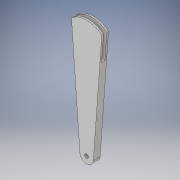
# Autodesk Inventor part: poker
Saved by Autodesk Inventor 2018 (Build 220112000, 112)
## iProperties
Created: 2017-12-11
Part Number: poker
Material: Generic
Document SubType Name: Modeling
Designer: ragna
Density: 1 g/cm^3
Appearance: Default
Author: ragna
Autodesk Inventor part; units mm, degrees
ref_plane "YZ Plane" through (0, 0, 0) normal (1, 0, 0) x (0, 1, 0)
ref_plane "XZ Plane" through (0, 0, 0) normal (0, 1, 0) x (-1, 0, 0)
ref_plane "XY Plane" through (0, 0, 0) normal (0, 0, 1) x (1, 0, 0)
sketch "Sketch1" plane through (0, 0, 0) normal (0, 0, 1) x (1, 0, 0)
  arc A0 (-0.1732, -0.9119) -> (-5.8268, -0.9119) centre (-3, -4.8375) ccw
  arc A1 (-5.8268, -1.5881) -> (-0.1732, -1.5881) centre (-3, 2.3375) ccw
  circle A2 centre (-5.5833, -1.25) radius 0.4167
  circle A3 centre (-0.4167, -1.25) radius 0.4167
  line L0 (-6, 0) -> (0, 0)
  line L1 (0, 0) -> (0, -2.5)
  line L2 (0, -2.5) -> (-6, -2.5)
  line L3 (-6, -2.5) -> (-6, 0)
  point P0 (-1.5, -3.25)
  dimension "d8" = 4.8375
  dimension "d11" = 0.8333
  dimension "d12" = 6
  dimension "d13" = 2.5
  dimension "d14" = 0.8333
  dimension "d22" = 4.8375
  constraints: 8 end point, 8 point on circle, 8 tangent, 4 centre point, 2 parallel, 1 coincident, 1 horizontal, 1 perpendicular, 1 vertical alignment
  measures "d8" radius of A0
  measures "d11" diameter of A3
  measures "d12" distance of L1.end L2.end
  measures "d13" distance of L2.end L0.start
  measures "d14" diameter of A2
  measures "d22" radius of A1
extrude "Extrusion1" add sketch "Sketch1" against normal blind 0.25 contours A3 A1 A2 A0 | A3 | A2
sketch "Sketch2" plane through (0, 0, 0) normal (0, 0, 1) x (1, 0, 0)
  arc A0 (-0.1732, -0.9119) -> (-5.8268, -0.9119) centre (-3, -4.8375) ccw projected
  arc A1 (1.5, 0.3105) -> (-7.5, 0.3105) centre (-3, -4.8375) ccw
  line L0 (-4.9944, -33.1493) -> (-7.5, 0.3105)
  line L1 (-1.0056, -33.1493) -> (1.5, 0.3105)
  circle A2 centre (-3, -33) radius 2
  arc A3 (-0.1732, -0.9119) -> (-5.8268, -0.9119) centre (-3, -4.8375) ccw projected
  line L2 (-11.9492, 2) -> (-1.5879, 2) construction
  point P0 (-7.5, -3.25)
  dimension "d15" = 33.5535
  dimension "d16" = 2
  dimension "d17" = 33.5535
  dimension "d19" = 4
  dimension "d20" = 9
  dimension "d21" = 35
  constraints: 6 end point, 4 point on circle, 3 tangent, 2 centre point, 1 horizontal, 1 vertical alignment, 1 other
  measures "d15" distance of L0.start L0.end
  measures "d17" distance of L1.start L1.end
  measures "d19" diameter of A2
  measures "d20" distance of L1.end L0.end
  measures "d21" distance from line of L2 A2.centre
extrude "Extrusion2" add sketch "Sketch2" along normal blind 0.5
sketch "Sketch4" plane through (0, 0, 0) normal (0, 0, -1) x (-1, 0, 0)
  arc A0 (7.5, 0.3105) -> (-1.5, 0.3105) centre (3, -4.8375) ccw projected
  line L0 (4.6338, -2.5) -> (0.9036, -2.5) construction
  line L1 (4.4698, -6) -> (1.0404, -6) construction
  arc A1 (0.1732, -1.5881) -> (5.8268, -1.5881) centre (3, 2.3375) ccw construction
  line L2 (7.5, 0.3105) -> (4.9944, -33.1493) construction
  line L3 (1.0056, -33.1493) -> (-1.5, 0.3105) construction
  arc A2 (6.9342, -7.2452) -> (-0.9342, -7.2452) centre (3, -12.8375) ccw
  line L4 (7.5, 0.3105) -> (4.9944, -33.1493) construction
  line L5 (1.0056, -33.1493) -> (-1.5, 0.3105) construction
  arc A3 (1.0056, -33.1493) -> (4.9944, -33.1493) centre (3, -33) ccw projected
  line L6 (6.9342, -7.2452) -> (4.9944, -33.1493)
  line L7 (1.0056, -33.1493) -> (-0.9342, -7.2452)
  point P0 (0, 0)
  dimension "d23" = 3.5
  dimension "d24" = 6.8375
  dimension "d25" = 6.8375
  constraints: 8 end point, 3 point on circle, 3 tangent, 2 collinear, 2 horizontal, 2 point on line, 1 centre point, 1 horizontal alignment
  measures "d23" distance between parallel lines of L0 L1
  measures "d24" radius of A2
  measures "d25" radius of A0
extrude "Extrusion4" add sketch "Sketch4" along normal blind 0.5
sketch "Sketch3" plane through (0, 0, 0.5) normal (0, 0, 1) x (1, 0, 0)
  arc A0 (-4.9944, -33.1493) -> (-1.0056, -33.1493) centre (-3, -33) ccw projected
  circle A1 centre (-3, -33) radius 0.55
  point P0 (0, 0)
  dimension "d5" = 1.1
  constraints: 1 centre point, 1 coincident
  measures "d5" diameter of A1
extrude "Extrusion3" cut sketch "Sketch3" against normal through all
mirror "Mirror1" about plane through (-3, -19.8277, -0.5) normal (0, 0, -1) of "Extrusion1", "Extrusion2", "Extrusion4", "Extrusion3"
sketch "Sketch6" plane through (-3, -4.8375, -1.5) normal (0, 0, -1) x (-1, 0, 0)
  line L0 (-1.9944, -28.3118) -> (-4.5, 5.148) projected
  line L1 (4.5, 5.148) -> (1.9944, -28.3118) projected
  arc A0 (-2.5219, -21.2673) -> (2.5219, -21.2673) centre (0, -18.1625) ccw
  circle A1 centre (0, -28.1625) radius 0.55 projected
  arc A2 (-1.9944, -28.3118) -> (1.9944, -28.3118) centre (0, -28.1625) ccw projected
  point P0 (-3, 4.8375)
  dimension "d31" = 4
  dimension "d32" = 10
  constraints: 2 point on circle, 2 point on line, 1 centre point, 1 horizontal alignment
  measures "d31" radius of A0
  measures "d32" distance of A1.centre A0.centre
equation "\"d11\" = 0.333333 * d13"
equation "\"d12\" = phheight"
equation "\"d13\" = phwidth"
equation "\"d14\" = d11"
equation "\"d22\" = d8"
equation "\"d16\" = phtosolid"
equation "\"d17\" = d15"
equation "\"d20\" = pheight"
equation "\"d24\" = d25"
equation "\"phheight\" = 6"
equation "\"phwidth\" = 2.5"
equation "\"phtosolid\" = 2"
equation "\"pheight\" = 9"
body "Solid1"
